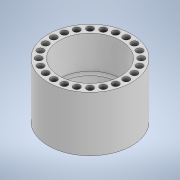
# Autodesk Inventor part: Kolo
Saved by Autodesk Inventor 2020 (Build 240168000, 168)
## iProperties
Created: 2019-12-20
Part Number: Kolo
Material: Generic
Document SubType Name: Modeling
Designer: atmat
Density: 1 g/cm^3
Appearance: Default
Author: atmat
Autodesk Inventor part; units mm, degrees
ref_plane "YZ Plane" through (0, 0, 0) normal (1, 0, 0) x (0, 1, 0)
ref_plane "XZ Plane" through (0, 0, 0) normal (0, 1, 0) x (-1, 0, 0)
ref_plane "XY Plane" through (0, 0, 0) normal (0, 0, 1) x (1, 0, 0)
sketch "Sketch1" plane through (0, 0, 0) normal (0, 1, 0) x (-1, 0, 0)
  circle A0 centre (0, 0) radius 19
  circle A1 centre (0, 0) radius 14
  dimension "d0" = 38
  dimension "d1" = 28
  constraints: 2 centre point, 2 coincident
  measures "d0" diameter of A0
  measures "d1" diameter of A1
extrude "Extrusion1" add sketch "Sketch1" along normal blind 25
sketch "Sketch2" plane through (0, 25, 0) normal (0, 1, 0) x (1, 0, 0)
  circle A0 centre (0, -16.5) radius 1.5
  circle A1 centre (0, 0) radius 14 projected
  dimension "d4" = 3
  dimension "d5" = 16.5
  constraints: 1 centre point
  measures "d4" diameter of A0
  measures "d5" distance of A1.centre A0.centre
extrude "Extrusion2" cut sketch "Sketch2" against normal blind 25 contours A0
pattern_circular "Circular Pattern1" count 24 over 360 about axis through (0, -10, 0) along (0, 1, 0) of "Extrusion2"
sketch "Sketch3" plane through (0, 0, 0) normal (0, 1, 0) x (-1, 0, 0)
  circle A0 centre (0, 0) radius 14
  circle A1 centre (0, 0) radius 13
  dimension "d11" = 26
  constraints: 2 centre point, 2 coincident
  measures "d11" diameter of A1
extrude "Extrusion3" add sketch "Sketch3" along normal blind 10
chamfer "Chamfer1" distance 1 angle 45 1 edges at (13, 10, 0)
body "Solid1"
